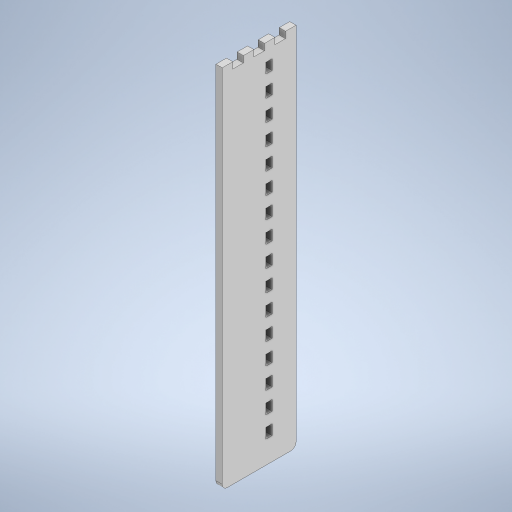
# Autodesk Inventor part: Module_supportZ_MFC
Saved by Autodesk Inventor 2023 (Build 270158000, 158)
## iProperties
Created: 2022-10-31
Part Number: Module_supportZ_MFC
Material: Generic
Document SubType Name: Modeling
Designer: incep
Density: 1 g/cm^3
Appearance: Default
Author: incep
Autodesk Inventor part; units mm, degrees
ref_plane "YZ Plane" through (0, 0, 0) normal (1, 0, 0) x (0, 1, 0)
ref_plane "XZ Plane" through (0, 0, 0) normal (0, 1, 0) x (-1, 0, 0)
ref_plane "XY Plane" through (0, 0, 0) normal (0, 0, 1) x (1, 0, 0)
sketch "Sketch1" plane through (0, 0, 0) normal (1, 0, 0) x (0, 1, 0)
  line L0 (0, 70) -> (-341.3, 70)
  line L1 (-341.3, 70) -> (-341.3, 0)
  line L2 (-341.3, 0) -> (0, 0)
  line L3 (0, 0) -> (0, 60) construction
  line L4 (0, 70) -> (6, 70)
  line L5 (6, 70) -> (6, 60)
  line L6 (6, 60) -> (0, 60)
  line L7 (0, 50) -> (6, 50)
  line L8 (6, 50) -> (6, 40)
  line L9 (6, 40) -> (0, 40)
  line L10 (0, 30) -> (6, 30)
  line L11 (6, 30) -> (6, 20)
  line L12 (6, 20) -> (0, 20)
  line L13 (0, 10) -> (6, 10)
  line L14 (6, 10) -> (6, 0)
  line L15 (6, 0) -> (0, 0)
  line L16 (0, 60) -> (0, 50)
  line L17 (0, 40) -> (0, 30)
  line L18 (0, 20) -> (0, 10)
  line L19 (-10.15, 28.525) -> (-19.85, 28.525)
  line L20 (-19.85, 28.525) -> (-19.85, 22.675)
  line L21 (-19.85, 22.675) -> (-10.15, 22.675)
  line L22 (-10.15, 22.675) -> (-10.15, 28.525)
  line L23 (-10, 28.6) -> (-331.3, 28.6) construction
  line L24 (-331.3, 28.6) -> (-331.3, 22.6) construction
  line L25 (-331.3, 22.6) -> (-10, 22.6) construction
  line L26 (-10, 22.6) -> (-10, 28.6) construction
  line L27 (-15, 28.6) -> (-15, 22.6) construction
  line L28 (-30.15, 22.675) -> (-30.15, 28.525)
  line L29 (-30.15, 28.525) -> (-39.85, 28.525)
  line L30 (-39.85, 22.675) -> (-30.15, 22.675)
  line L31 (-39.85, 28.525) -> (-39.85, 22.675)
  line L32 (-50.15, 22.675) -> (-50.15, 28.525)
  line L33 (-50.15, 28.525) -> (-59.85, 28.525)
  line L34 (-59.85, 22.675) -> (-50.15, 22.675)
  line L35 (-59.85, 28.525) -> (-59.85, 22.675)
  line L36 (-70.15, 22.675) -> (-70.15, 28.525)
  line L37 (-70.15, 28.525) -> (-79.85, 28.525)
  line L38 (-79.85, 22.675) -> (-70.15, 22.675)
  line L39 (-79.85, 28.525) -> (-79.85, 22.675)
  line L40 (-90.15, 22.675) -> (-90.15, 28.525)
  line L41 (-90.15, 28.525) -> (-99.85, 28.525)
  line L42 (-99.85, 22.675) -> (-90.15, 22.675)
  line L43 (-99.85, 28.525) -> (-99.85, 22.675)
  line L44 (-110.15, 22.675) -> (-110.15, 28.525)
  line L45 (-110.15, 28.525) -> (-119.85, 28.525)
  line L46 (-119.85, 22.675) -> (-110.15, 22.675)
  line L47 (-119.85, 28.525) -> (-119.85, 22.675)
  line L48 (-130.15, 22.675) -> (-130.15, 28.525)
  line L49 (-130.15, 28.525) -> (-139.85, 28.525)
  line L50 (-139.85, 22.675) -> (-130.15, 22.675)
  line L51 (-139.85, 28.525) -> (-139.85, 22.675)
  line L52 (-150.15, 22.675) -> (-150.15, 28.525)
  line L53 (-150.15, 28.525) -> (-159.85, 28.525)
  line L54 (-159.85, 22.675) -> (-150.15, 22.675)
  line L55 (-159.85, 28.525) -> (-159.85, 22.675)
  line L56 (-170.15, 22.675) -> (-170.15, 28.525)
  line L57 (-170.15, 28.525) -> (-179.85, 28.525)
  line L58 (-179.85, 22.675) -> (-170.15, 22.675)
  line L59 (-179.85, 28.525) -> (-179.85, 22.675)
  line L60 (-190.15, 22.675) -> (-190.15, 28.525)
  line L61 (-190.15, 28.525) -> (-199.85, 28.525)
  line L62 (-199.85, 22.675) -> (-190.15, 22.675)
  line L63 (-199.85, 28.525) -> (-199.85, 22.675)
  line L64 (-210.15, 22.675) -> (-210.15, 28.525)
  line L65 (-210.15, 28.525) -> (-219.85, 28.525)
  line L66 (-219.85, 22.675) -> (-210.15, 22.675)
  line L67 (-219.85, 28.525) -> (-219.85, 22.675)
  line L68 (-230.15, 22.675) -> (-230.15, 28.525)
  line L69 (-230.15, 28.525) -> (-239.85, 28.525)
  line L70 (-239.85, 22.675) -> (-230.15, 22.675)
  line L71 (-239.85, 28.525) -> (-239.85, 22.675)
  line L72 (-250.15, 22.675) -> (-250.15, 28.525)
  line L73 (-250.15, 28.525) -> (-259.85, 28.525)
  line L74 (-259.85, 22.675) -> (-250.15, 22.675)
  line L75 (-259.85, 28.525) -> (-259.85, 22.675)
  line L76 (-270.15, 22.675) -> (-270.15, 28.525)
  line L77 (-270.15, 28.525) -> (-279.85, 28.525)
  line L78 (-279.85, 22.675) -> (-270.15, 22.675)
  line L79 (-279.85, 28.525) -> (-279.85, 22.675)
  line L80 (-290.15, 22.675) -> (-290.15, 28.525)
  line L81 (-290.15, 28.525) -> (-299.85, 28.525)
  line L82 (-299.85, 22.675) -> (-290.15, 22.675)
  line L83 (-299.85, 28.525) -> (-299.85, 22.675)
  line L84 (-310.15, 22.675) -> (-310.15, 28.525)
  line L85 (-310.15, 28.525) -> (-319.85, 28.525)
  line L86 (-319.85, 22.675) -> (-310.15, 22.675)
  line L87 (-319.85, 28.525) -> (-319.85, 22.675)
  point P0 (0, 35)
  point P1 (-170.65, 0)
  point P2 (3, 70)
  point P3 (3, 50)
  point P4 (3, 30)
  point P5 (3, 10)
  point P6 (-10.15, 25.6)
  point P7 (-10, 25.6)
  point P8 (0, 35)
  point P9 (-15, 25.6)
  point P10 (-15, 22.675)
  point P11 (-30.15, 25.6)
  point P12 (-35, 22.675)
  point P13 (-50.15, 25.6)
  point P14 (-55, 22.675)
  point P15 (-70.15, 25.6)
  point P16 (-75, 22.675)
  point P17 (-90.15, 25.6)
  point P18 (-95, 22.675)
  point P19 (-110.15, 25.6)
  point P20 (-115, 22.675)
  point P21 (-130.15, 25.6)
  point P22 (-135, 22.675)
  point P23 (-150.15, 25.6)
  point P24 (-155, 22.675)
  point P25 (-170.15, 25.6)
  point P26 (-175, 22.675)
  point P27 (-190.15, 25.6)
  point P28 (-195, 22.675)
  point P29 (-210.15, 25.6)
  point P30 (-215, 22.675)
  point P31 (-230.15, 25.6)
  point P32 (-235, 22.675)
  point P33 (-250.15, 25.6)
  point P34 (-255, 22.675)
  point P35 (-270.15, 25.6)
  point P36 (-275, 22.675)
  point P37 (-290.15, 25.6)
  point P38 (-295, 22.675)
  point P39 (-310.15, 25.6)
  point P40 (-315, 22.675)
  dimension "d7" = 70
  dimension "d18" = 6
  dimension "d21" = 10
  dimension "d24" = 341.3
  dimension "d35" = 20
  dimension "d49" = 5.85
  dimension "d50" = 9.7
  dimension "d51" = 6
  dimension "d52" = 9.4
  dimension "d53" = 10
  dimension "d58" = 10
  dimension "d60" = 5
  dimension "d63" = 20
  constraints: 176 end point, 7 midpoint, 7 parallel, 5 horizontal, 5 perpendicular, 3 collinear, 3 point on line, 2 horizontal alignment, 2 vertical alignment, 1 vertical, 174 other
  measures "d7" distance between parallel lines of L2 L0
  measures "d18" distance of L3.end L5.end
  measures "d21" distance of L4.end L5.end
  measures "d24" distance between parallel lines of L1 L3
  measures "d35" distance of L0.start L7.start
  measures "d49" distance between parallel lines of L21 L19
  measures "d50" distance from line of L20 point (-10.15, 25.6)
  measures "d51" distance between parallel lines of L25 L23
  measures "d52" vertical distance of point (-10, 25.6) point (0, 35)
  measures "d53" distance from line of point (0, 35) L26
  measures "d58" distance between parallel lines of L1 L24
  measures "d60" distance from line of L26 point (-15, 25.6)
  measures "d63" distance of L21.end L28.start
extrude "Extrusion1" add sketch "Sketch1" along normal blind 6
fillet "Fillet1" radius 5 2 edges at (3, -341.3, 70) (3, -341.3, 0)
equation "\"d7\" = moduleMountH"
equation "\"d18\" = fingerH"
equation "\"d21\" = fingerW"
equation "\"d24\" = supportL"
equation "\"d35\" = fingerSpacing"
equation "\"d49\" = fingerholeH"
equation "\"d50\" = fingerholeW"
equation "\"d51\" = thickness"
equation "\"d52\" = supportsCTCZ"
equation "\"d53\" = 0.5 * fingerSpacing"
equation "\"d58\" = 0.5 * fingerSpacing"
equation "\"d60\" = 0.5 * fingerW"
equation "\"d63\" = fingerSpacing"
equation "\"d44\" = thickness"
equation "\"d73\" = supportsFilletR"
equation "\"moduleWidth\" = 118"
equation "\"moduleHeight\" = 96"
equation "\"moduleMountH\" = 70"
equation "\"moduleMountD\" = 6.8"
equation "\"moduleCornerR\" = 5"
equation "\"d4\" = moduleCornerR"
equation "\"d5\" = moduleMountD"
equation "\"d6\" = moduleMountD"
equation "\"d8\" = moduleMountD"
equation "\"d10\" = moduleMountD"
equation "\"moduleOpeningR\" = 25"
equation "\"d13\" = moduleOpeningR"
equation "\"thickness\" = 6"
equation "\"d15\" = thickness"
equation "\"d16\" = 0"
equation "\"kerf\" = 0.15"
equation "\"fingerW\" = 10"
equation "\"fingerSpacing\" = 20"
equation "\"fingerholeW\" = fingerW - 2 * kerf"
equation "\"fingerholeH\" = thickness - kerf"
equation "\"moduleMountClearance\" = 19"
equation "\"actuatorW\" = 28"
equation "\"actuatorH\" = 40.8"
equation "\"openingMFC\" = 45"
equation "\"d28\" = thickness"
equation "\"d29\" = thickness"
equation "\"d30\" = 0.5 * actuatorH + thickness"
equation "\"d31\" = 15"
equation "\"d32\" = fingerholeH"
equation "\"d33\" = fingerholeW"
equation "\"d41\" = fingerholeH"
equation "\"d42\" = fingerholeW"
equation "\"chairThickness\" = 12.7"
equation "\"supportL\" = -chairThickness + dildoL + actuatorMountL - thickness"
equation "\"d0\" = moduleHeight"
equation "\"d1\" = moduleWidth"
equation "\"d17\" = openingMFC"
equation "\"d19\" = moduleMountClearance"
equation "\"fingerH\" = thickness"
equation "\"supportSpacingFromMounting\" = 15"
equation "\"d54\" = fingerholeH"
equation "\"d55\" = fingerholeW"
equation "\"d64\" = 9.4"
equation "\"supportsCTCZ\" = d64"
equation "\"supportXW\" = -2 * thickness + moduleMountW - 2 * supportSpacingFromMounting + kerf"
equation "\"supportsFilletR\" = 5"
equation "\"dildoL\" = 170"
equation "\"actuatorMountL\" = 190"
equation "\"moduleMountW\" = 100"
body "Solid1"
